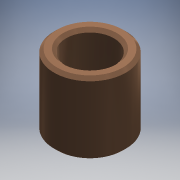
# Autodesk Inventor part: BearingBronze8x12x12
Saved by Autodesk Inventor 2016 (Build 200138000, 138)
## iProperties
Created: 2015-05-21
Part Number: BearingBronze8x12x12
Material: Bronze, Cast
Document SubType Name: Modeling
Designer: Jack
Density: 8.87 g/cm^3
Appearance: Bronze - Satin
Author: Jack
Autodesk Inventor part; units mm, degrees
ref_plane "YZ Plane" through (0, 0, 0) normal (1, 0, 0) x (0, 1, 0)
ref_plane "XZ Plane" through (0, 0, 0) normal (0, 1, 0) x (-1, 0, 0)
ref_plane "XY Plane" through (0, 0, 0) normal (0, 0, 1) x (1, 0, 0)
sketch "Sketch1" plane through (0, 0, 0) normal (0, 0, 1) x (1, 0, 0)
  circle A0 centre (0, 0) radius 4
  circle A1 centre (0, 0) radius 6
  dimension "d0" = 12
  dimension "d1" = 8
  constraints: 2 centre point, 2 coincident
  measures "d0" diameter of A1
  measures "d1" diameter of A0
extrude "Extrusion1" add sketch "Sketch1" along normal blind 12
chamfer "Chamfer1" distance 0.5 angle 45 4 edges at (-6, 0, 12) (-6, 0, 0) (-4, 0, 12) (-4, 0, 0)
body "Solid1"
